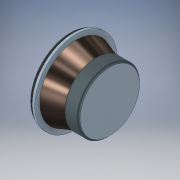
# Autodesk Inventor part: Loudspeaker
Saved by Autodesk Inventor 2018.3 (Build 223284000, 284)
## iProperties
Created: 2018-06-03
Part Number: Loudspeaker
Material: Generisch
Document SubType Name: Modeling
Designer: JochenAlt
Density: 1 g/cm^3
Appearance: Stahlblau
Author: JochenAlt
Autodesk Inventor part; units mm, degrees
ref_plane "YZ Plane" through (0, 0, 0) normal (1, 0, 0) x (0, 1, 0)
ref_plane "XZ Plane" through (0, 0, 0) normal (0, 1, 0) x (-1, 0, 0)
ref_plane "XY Plane" through (0, 0, 0) normal (0, 0, 1) x (1, 0, 0)
sketch "Skizze1" plane through (0, 0, 0) normal (0, 1, 0) x (-1, 0, 0)
  line L0 (39.8687, 22.5) -> (39.8687, 24)
  line L1 (39.8687, 24) -> (37.8687, 24)
  line L2 (37.8687, 24) -> (37.8687, 25)
  line L3 (37.8687, 25) -> (36.3687, 25)
  line L4 (36.3687, 22) -> (24.8687, 18.0718)
  line L5 (24.8687, 18.0718) -> (24.8687, 17.0718)
  line L6 (24.8687, 17.0718) -> (23.8687, 17.0718)
  line L7 (23.8687, 17.0718) -> (23.8687, 19)
  line L8 (23.8687, 19) -> (16.8687, 19)
  line L9 (16.8687, 19) -> (16.8687, 18)
  line L10 (16.8687, 18) -> (15.8687, 18)
  line L11 (15.8687, 18) -> (15.8687, 0)
  line L12 (39.8687, 22.5) -> (37.3687, 22.5)
  arc A0 (37.3687, 18.5) -> (37.3687, 22.5) centre (37.3687, 20.5) ccw
  line L13 (37.3687, 18.5) -> (30.1519, 6)
  arc A1 (32.1519, 0) -> (30.1519, 6) centre (22.1519, 0) ccw
  line L14 (0, -5) -> (0, 30) construction
  line L15 (-7.9737, 0) -> (47.8425, 0) construction
  line L16 (37.3687, 22.5) -> (37.3687, 18.5) construction
  line L17 (32.1519, 0) -> (15.8687, 0)
  line L18 (36.3687, 25) -> (36.3687, 22)
  point P0 (0, 0)
  dimension "d1" = 2
  dimension "d2" = 30
  dimension "d3" = 6
  dimension "d4" = 22.5
  dimension "d5" = 24
  dimension "d6" = 2
  dimension "d7" = 1
  dimension "d8" = 24
  dimension "d10" = 18
  dimension "d11" = 7
  dimension "d13" = 1
  dimension "d14" = 1
  dimension "d16" = 1
  dimension "d17" = 1.5
  dimension "d18" = 2
  dimension "d19" = 2.5
  dimension "d20" = 1
  dimension "d23" = 3
  constraints: 34 end point, 9 perpendicular, 4 point on circle, 2 centre point, 2 horizontal, 2 point on line, 2 vertical, 1 collinear, 1 line through centre, 1 midpoint, 1 parallel
  measures "d1" radius of A0
  measures "d2" angle of L14 L13
  measures "d3" distance from line of L15 L13.end
  measures "d4" distance between parallel lines of L15 L12
  measures "d5" distance between parallel lines of L15 L1
  measures "d6" distance between parallel lines of L2 L0
  measures "d7" distance of L1.end L2.end
  measures "d8" distance between parallel lines of L11 L0
  measures "d10" distance of L10.end L11.end
  measures "d11" distance of L7.end L8.end
  measures "d13" distance of L9.end L10.end
  measures "d14" distance of L5.end L6.end
  measures "d16" distance of L8.end L9.end
  measures "d17" distance of L2.end L3.end
  measures "d18" horizontal distance of L17.start L13.end
  measures "d19" distance of L0.start L12.end
  measures "d20" distance of L4.end L5.end
  measures "d23" distance of L3.end L4.start
revolve "Umdrehung1" add sketch "Skizze1" angle 360 about axis through (0, 0, 0) along (-1, 0, 0)
